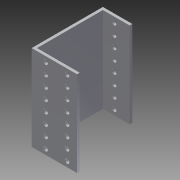
# Autodesk Inventor part: Chass_EndCaps
Saved by Autodesk Inventor 2014 (Build 180170000, 170)
## iProperties
Created: 2016-01-25
Part Number: Chass_EndCaps
Material: Aluminum 6061
Document SubType Name: Modeling
Designer: choices
Density: 2.71 g/cm^3
Appearance: Aluminum - Flat
Author: choices
Autodesk Inventor part; units mm, degrees
ref_plane "YZ Plane" through (0, 0, 0) normal (1, 0, 0) x (0, 1, 0)
ref_plane "XZ Plane" through (0, 0, 0) normal (0, 1, 0) x (-1, 0, 0)
ref_plane "XY Plane" through (0, 0, 0) normal (0, 0, 1) x (1, 0, 0)
sketch "Sketch1" plane through (0, 0, 0) normal (0, 1, 0) x (-1, 0, 0)
  line L0 (-3.4862, 4.6259) -> (50.4888, 4.6259)
  line L1 (50.4888, 4.6259) -> (50.4888, -79.9561)
  line L2 (50.4888, -79.9561) -> (-3.4862, -79.9561)
  line L3 (-3.4862, 1.4509) -> (-3.4862, 4.6259)
  line L4 (-3.4862, 1.4509) -> (47.3138, 1.4509)
  line L5 (47.3138, 1.4509) -> (47.3138, -76.7811)
  line L6 (47.3138, -76.7811) -> (15.5638, -76.7811)
  line L7 (15.5638, -76.7811) -> (15.5638, -79.9561)
  point P0 (0, 0)
  dimension "d0" = 53.975
  dimension "d1" = 84.582
  dimension "d2" = 3.175
  dimension "d3" = 50.8
  dimension "d4" = 78.232
  dimension "d5" = 31.75
  constraints: 16 end point, 5 perpendicular, 2 parallel, 1 horizontal, 1 point on line
  measures "d0" distance of L1.end L2.end
  measures "d1" distance of L0.end L1.end
  measures "d2" distance from line of L3.start L0
  measures "d3" distance of L3.start L4.end
  measures "d4" distance of L4.end L5.end
  measures "d5" distance of L5.end L6.end
extrude "Extrusion1" add sketch "Sketch1" along normal blind 101.6
sketch "Sketch2" plane through (-50.4888, 0, 4.6259) normal (0, 0, 1) x (1, 0, 0)
  line L0 (0, 101.6) -> (53.975, 101.6) projected
  line L1 (0, 0) -> (0, 101.6) projected
  circle A0 centre (16.637, 95.25) radius 2.667
  circle A1 centre (42.037, 95.25) radius 2.6686
  circle A2 centre (16.637, 82.55) radius 2.667
  circle A3 centre (42.037, 82.55) radius 2.6686
  circle A4 centre (16.637, 69.85) radius 2.667
  circle A5 centre (42.037, 69.85) radius 2.6686
  circle A6 centre (16.637, 57.15) radius 2.667
  circle A7 centre (42.037, 57.15) radius 2.6686
  circle A8 centre (16.637, 44.45) radius 2.667
  circle A9 centre (42.037, 44.45) radius 2.6686
  circle A10 centre (16.637, 31.75) radius 2.667
  circle A11 centre (42.037, 31.75) radius 2.6686
  circle A12 centre (16.637, 19.05) radius 2.667
  circle A13 centre (42.037, 19.05) radius 2.6686
  circle A14 centre (16.637, 6.35) radius 2.667
  circle A15 centre (42.037, 6.35) radius 2.6686
  point P0 (50.4888, 0)
  dimension "d8" = 5.334
  dimension "d9" = 6.35
  dimension "d10" = 16.637
  dimension "d11" = 25.4
  dimension "d14" = 12.7
  constraints: 16 centre point, 1 vertical, 28 other
  measures "d8" diameter of A0
  measures "d9" distance from line of L0 A0.centre
  measures "d10" distance from line of L1 A0.centre
  measures "d11" distance of A1.centre A0.centre
  measures "d14" distance of A0.centre A2.centre
extrude "Extrusion2" cut sketch "Sketch2" against normal blind 104.775
body "Solid1"
